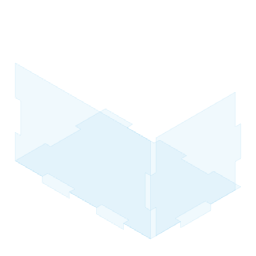
box v0 (Autodesk Fusion 360 design; units mm, degrees)
Autodesk Fusion 360 part; units mm, degrees
sketch "Base " plane through (0, 0, 0) normal (0, 0, 1) x (1, 0, 0)
  line L0 (0, 0) -> (75, 0)
  line L1 (75, 0) -> (75, 50)
  line L2 (75, 50) -> (0, 50)
  line L3 (0, 50) -> (0, 0)
  dimension "d8" = 75
  dimension "d9" = 50
  constraint horizontal L0
  constraint vertical L1
  constraint horizontal L2
  constraint vertical L3
  constraint coincident L0.start L3.end
  measures "d8" distance of L0.start L0.end
  measures "d9" distance of L0.end L1.end
extrude "Extrude1" add sketch "Base " along normal blind 3 makes body 1
sketch "Sketch3" plane through (0, 0, 0) normal (0, -1, 0) x (1, 0, 0)
  line L0 (0, 0) -> (75, 0)
  line L1 (75, 0) -> (75, 3)
  line L2 (75, 3) -> (0, 3)
  line L3 (0, 3) -> (0, 0)
  line L4 (0, 0) -> (75, 0)
  line L5 (75, 0) -> (75, 50)
  line L6 (75, 50) -> (0, 50)
  line L7 (0, 50) -> (0, 0)
  dimension "d12" = 50
  constraint horizontal L4
  constraint vertical L5
  constraint horizontal L6
  constraint vertical L7
  constraint coincident L0.start L3.end
  measures "d12" distance of L4 L6
sketch "Sketch4" plane through (0, 0, 0) normal (0, -1, 0) x (1, 0, 0)
  line L0 (0, 50) -> (0, 0)
  line L1 (75, 0) -> (75, 50)
  line L2 (15, 0) -> (30, 0)
  line L3 (30, 0) -> (30, 3)
  line L4 (30, 3) -> (15, 3)
  line L5 (15, 3) -> (15, 0)
  line L6 (45, 0) -> (60, 0)
  line L7 (60, 0) -> (60, 3)
  line L8 (60, 3) -> (45, 3)
  line L9 (45, 3) -> (45, 0)
  dimension "d19" = 15
  dimension "d20" = 15
  dimension "d21" = 15
  dimension "d22" = 15
  constraint horizontal L2
  constraint vertical L3
  constraint horizontal L4
  constraint vertical L5
  constraint horizontal L6
  constraint vertical L7
  constraint horizontal L8
  constraint vertical L9
  measures "d19" distance of L3 L5
  measures "d20" distance of L3 L9
  measures "d21" distance of L7 L9
  measures "d22" distance of L0 L5
extrude "Extrude2" add sketch "Sketch3" sketch "Sketch4" against normal blind 3 separate body contours L2 L5 L6 L7 of sketch 2 makes body 2
extrude "Extrude3" add 1 faces at (40, 0, 34.3333) along direction (0, -1, 0) blind 3 from surface at -50 separate body on bodies 2 makes body 3
combine "Combine1" operation cut target body 1 tool bodies 3 2 keep tools
sketch "Sketch5" plane through (75, 0, 0) normal (1, 0, 0) x (0, 1, 0)
  line L0 (0, 0) -> (50, 0)
  line L1 (50, 0) -> (50, 3)
  line L2 (50, 3) -> (0, 3)
  line L3 (0, 3) -> (0, 0)
  line L4 (0, 50) -> (0, 3)
  line L5 (0, 3) -> (3, 3)
  line L6 (3, 3) -> (3, 50)
  line L7 (3, 50) -> (0, 50)
  line L8 (50, 3) -> (50, 50)
  line L9 (50, 50) -> (47, 50)
  line L10 (47, 50) -> (47, 3)
  line L11 (47, 3) -> (50, 3)
  line L12 (0, 0) -> (50, 0)
  line L13 (50, 0) -> (50, 50)
  line L14 (50, 50) -> (0, 50)
  line L15 (0, 50) -> (0, 0)
  line L16 (16.6667, 0) -> (33.3333, 0)
  line L17 (33.3333, 0) -> (33.3333, 3)
  line L18 (33.3333, 3) -> (16.6667, 3)
  line L19 (16.6667, 3) -> (16.6667, 0)
  line L20 (50, 33.3333) -> (47, 33.3333)
  line L21 (47, 33.3333) -> (47, 16.6667)
  line L22 (47, 16.6667) -> (50, 16.6667)
  line L23 (50, 16.6667) -> (50, 33.3333)
  line L24 (0, 33.3333) -> (3, 33.3333)
  line L25 (3, 33.3333) -> (3, 16.6667)
  line L26 (3, 16.6667) -> (0, 16.6667)
  line L27 (0, 16.6667) -> (0, 33.3333)
  dimension "d28" = 16.6667
  dimension "d29" = 16.6667
  dimension "d30" = 16.6667
  dimension "d31" = 16.6667
  dimension "d32" = 16.6667
  dimension "d33" = 16.6667
  constraint horizontal L12
  constraint vertical L13
  constraint horizontal L14
  constraint vertical L15
  constraint coincident L8.end L9.start
  constraint coincident L0.start L3.end
  constraint horizontal L16
  constraint vertical L17
  constraint horizontal L18
  constraint vertical L19
  constraint coincident L2 L17.end
  constraint coincident L12 L16.start
  constraint horizontal L20
  constraint vertical L21
  constraint horizontal L22
  constraint vertical L23
  constraint coincident L10 L21.end
  constraint coincident L8 L20.start
  constraint horizontal L24
  constraint vertical L25
  constraint horizontal L26
  constraint vertical L27
  constraint coincident L6 L25.end
  constraint coincident L15 L24.start
  measures "d28" distance of L14 L24
  measures "d29" distance of L24 L26
  measures "d30" distance of L17 L19
  measures "d31" distance of L13 L17
  measures "d32" distance of L14 L20
  measures "d33" distance of L20.end L21.end
extrude "Extrude4" add sketch "Sketch5" against normal blind 3 separate body contours L0 L2 L12 L16 L17 L18 L19 | L2 L6 L10 L14 L18 L21 L25 | L4 L6 L15 L24 L25 L26 L27 | L8 L10 L13 L20 L21 L22 L23 makes body 4
extrude "Extrude5" add 1 faces at (72, 27.7778, 23.2222) along direction (1, 0, 0) blind 3 from surface at -72 separate body on bodies 4 makes body 5
combine "Combine2" operation cut target body 1 tool bodies 5 4 keep tools
combine "Combine3" operation cut target body 2 tool bodies 5 4 keep tools
combine "Combine4" operation cut target body 3 tool bodies 5 4 keep tools
sketch "base dxf" plane through (0, 0, 3) normal (0, 0, 1) x (-1, 0, 0)
  line L0 (-75, -33.3333) -> (-75, -50)
  line L1 (-75, -50) -> (-60, -50)
  line L2 (-60, -50) -> (-60, -47)
  line L3 (-60, -47) -> (-45, -47)
  line L4 (-45, -47) -> (-45, -50)
  line L5 (-45, -50) -> (-30, -50)
  line L6 (-30, -50) -> (-30, -47)
  line L7 (-30, -47) -> (-15, -47)
  line L8 (-15, -47) -> (-15, -50)
  line L9 (-15, -50) -> (0, -50)
  line L10 (0, -50) -> (0, -33.3333)
  line L11 (0, -33.3333) -> (-3, -33.3333)
  line L12 (-3, -33.3333) -> (-3, -16.6667)
  line L13 (-3, -16.6667) -> (0, -16.6667)
  line L14 (0, -16.6667) -> (0, 0)
  line L15 (0, 0) -> (-15, 0)
  line L16 (-15, 0) -> (-15, -3)
  line L17 (-15, -3) -> (-30, -3)
  line L18 (-30, -3) -> (-30, 0)
  line L19 (-30, 0) -> (-45, 0)
  line L20 (-45, 0) -> (-45, -3)
  line L21 (-45, -3) -> (-60, -3)
  line L22 (-60, -3) -> (-60, 0)
  line L23 (-60, 0) -> (-75, 0)
  line L24 (-75, 0) -> (-75, -16.6667)
  line L25 (-75, -16.6667) -> (-72, -16.6667)
  line L26 (-72, -16.6667) -> (-72, -33.3333)
  line L27 (-72, -33.3333) -> (-75, -33.3333)
sketch "front dxf" plane through (0, 0, 0) normal (0, -1, 0) x (1, 0, 0)
  line L0 (72, 33.3333) -> (75, 33.3333)
  line L1 (75, 33.3333) -> (75, 50)
  line L2 (75, 50) -> (0, 50)
  line L3 (0, 50) -> (0, 33.3333)
  line L4 (0, 33.3333) -> (3, 33.3333)
  line L5 (3, 33.3333) -> (3, 16.6667)
  line L6 (3, 16.6667) -> (0, 16.6667)
  line L7 (0, 16.6667) -> (0, 3)
  line L8 (0, 3) -> (15, 3)
  line L9 (15, 3) -> (15, 0)
  line L10 (15, 0) -> (30, 0)
  line L11 (30, 0) -> (30, 3)
  line L12 (30, 3) -> (45, 3)
  line L13 (45, 3) -> (45, 0)
  line L14 (45, 0) -> (60, 0)
  line L15 (60, 0) -> (60, 3)
  line L16 (60, 3) -> (75, 3)
  line L17 (75, 3) -> (75, 16.6667)
  line L18 (75, 16.6667) -> (72, 16.6667)
  line L19 (72, 16.6667) -> (72, 33.3333)
sketch "side dxf" plane through (75, 0, 0) normal (1, 0, 0) x (0, 1, 0)
  line L0 (16.6667, 3) -> (16.6667, 0)
  line L1 (16.6667, 0) -> (33.3333, 0)
  line L2 (33.3333, 0) -> (33.3333, 3)
  line L3 (33.3333, 3) -> (47, 3)
  line L4 (47, 3) -> (47, 16.6667)
  line L5 (47, 16.6667) -> (50, 16.6667)
  line L6 (50, 16.6667) -> (50, 33.3333)
  line L7 (50, 33.3333) -> (47, 33.3333)
  line L8 (47, 33.3333) -> (47, 50)
  line L9 (47, 50) -> (3, 50)
  line L10 (3, 50) -> (3, 33.3333)
  line L11 (3, 33.3333) -> (0, 33.3333)
  line L12 (0, 33.3333) -> (0, 16.6667)
  line L13 (0, 16.6667) -> (3, 16.6667)
  line L14 (3, 16.6667) -> (3, 3)
  line L15 (3, 3) -> (16.6667, 3)
hidden bodies 1 2 3 4 5
equation "length = 75 mm" comment "box length"
equation "width = 50 mm" comment "box widtth"
equation "height = 50 mm" comment "box height"
equation "t = 3 mm" comment "thickness"
equation "slotL = length / 5" comment "length of tab @length"
equation "slotW = width / 3" comment "length of tab @width"
equation "slotH = height / 3" comment "length of tab @height"
equation "d8 = length"
equation "d9 = width"
equation "d10 = t"
equation "d12 = height"
equation "d19 = slotL"
equation "d20 = slotL"
equation "d21 = d20"
equation "d22 = d19"
equation "d23 = -t"
equation "d26 = t"
equation "d28 = slotH"
equation "d29 = d28"
equation "d30 = d29"
equation "d31 = d30"
equation "d32 = d29"
equation "d33 = d32"
equation "d34 = -t"
equation "d37 = -t"
named bodies: "Base"
